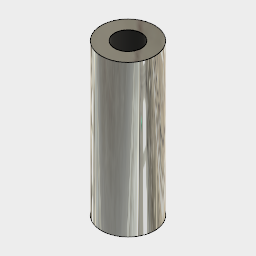
Print_Head_v5 (Autodesk Fusion 360 archive; units mm, degrees)
design "LM6LUU"
Autodesk Fusion 360 part; units mm, degrees
note: some values were not read from the file. Chosen so that the rebuilt part matches the saved one: which face or edge a step refers to. Set by a fixed rule: which sketch regions a step uses.
sketch "Sketch1" plane through (0, 0, 0) normal (0, 0, 1) x (1, 0, 0) in component "LM6LUU"
  circle A0 centre (0, 0) radius 6
  circle A1 centre (0, 0) radius 3
  dimension "d1" = 12
  dimension "d2" = 6
  measures "d1" diameter of A0
  measures "d2" diameter of A1
extrude "Extrude1" add sketch "Sketch1" along normal blind 34 makes body 1 in component "LM6LUU"
copy_body "CutPasteBodies1" bodies 1 removing the originals makes body 2 in component "LM6LUU"
component "LM6LUU" placed x (1, 0, 0) y (0, 1, 0) z (0, 0, 1) at (0, 0, 0)

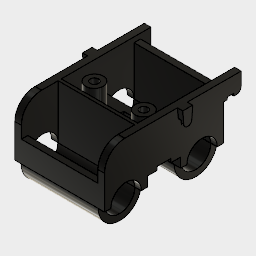
design "X Carriage"
Autodesk Fusion 360 part; units mm, degrees
sketch "Back" plane through (0, 0, 0) normal (0, 0, 1) x (1, 0, 0) in component "X Carriage"
  line L0 (17.75, 23.5) -> (-17.75, 23.5) construction
  line L1 (-17.75, 23.5) -> (-17.75, -23.5)
  line L2 (-17.75, -23.5) -> (17.75, -23.5)
  line L3 (17.75, -23.5) -> (17.75, 23.5)
  line L4 (0, 23.5) -> (0, -23.5) construction
  line L5 (-17.75, 23.5) -> (-17.75, 27.7)
  line L6 (-17.75, 27.7) -> (-15.1, 27.7)
  line L7 (17.75, 23.5) -> (17.75, 30.5)
  line L8 (17.75, 30.5) -> (15.1, 30.5)
  line L9 (15.1, 30.5) -> (15.1, 23.5)
  line L10 (-15.1, 27.7) -> (-15.1, 23.5)
  line L11 (-15.1, 23.5) -> (15.1, 23.5)
  line L12 (-15.1, 21) -> (15.1, 21)
  line L13 (15.1, 21) -> (15.1, -6.5)
  line L14 (15.1, -6.5) -> (-15.1, -6.5)
  line L15 (-15.1, -6.5) -> (-15.1, 21)
  line L16 (-15.1, -9) -> (15.1, -9)
  line L17 (15.1, -9) -> (15.1, -23.5)
  line L18 (-15.1, -9) -> (-15.1, -23.5)
  line L19 (15.1, -21) -> (-15.1, -21)
  line L20 (-9.75, 0) -> (9.75, 0) construction
  circle A0 centre (-9.75, 0) radius 1.6
  circle A1 centre (9.75, 0) radius 1.6
  circle A2 centre (-9.75, 0) radius 3.5
  circle A3 centre (9.75, 0) radius 3.5
  line L21 (15.1, -7.75) -> (-15.1, -7.75)
  line L22 (-15.1, -7.75) -> (-15.1, -6.5)
  line L23 (15.1, -7.75) -> (15.1, -6.5)
  line L24 (17.75, 9.2) -> (19.75, 9.2)
  line L25 (19.75, 9.2) -> (19.75, 5.3)
  line L26 (19.75, 5.3) -> (17.75, 5.3)
  line L27 (-17.75, 9.2) -> (-19.75, 9.2)
  line L28 (-19.75, 9.2) -> (-19.75, 5.3)
  line L29 (-19.75, 5.3) -> (-17.75, 5.3)
  line L30 (-4.5, -2.7) -> (4.5, -2.7)
  line L31 (4.5, -2.7) -> (4.5, 6.3)
  line L32 (4.5, 6.3) -> (-4.5, 6.3)
  line L33 (-4.5, 6.3) -> (-4.5, -2.7)
  line L34 (-3, -2.7) -> (-3, 3.3)
  line L35 (-3, 3.3) -> (3, 3.3)
  line L36 (3, 3.3) -> (3, -2.7)
  circle A4 centre (9.75, 0) radius 2.7
  circle A5 centre (-9.75, 0) radius 2.7
  line L37 (-15.1, 21) -> (-15.1, 23.5)
  line L38 (15.1, 21) -> (15.1, 23.5)
  line L39 (-15.1, 9) -> (15.1, 9)
  point P0 (0, 21)
  point P1 (0, -2.7)
  point P2 (0, 3.3)
  dimension "d1" = 35.5
  dimension "d2" = 47
  dimension "d3" = 4.2
  dimension "d5" = 7
  dimension "d7" = 30.2
  dimension "d8" = 27.5
  dimension "d9" = 2.5
  dimension "d10" = 2.5
  dimension "d11" = 2.5
  dimension "d12" = 19.5
  dimension "d13" = 3.2
  dimension "d14" = 3.2
  dimension "d15" = 7
  dimension "d16" = 7
  dimension "d17" = 21
  dimension "d18" = 1.25
  dimension "d20" = 3.9
  dimension "d21" = 2
  dimension "d22" = 28.8
  dimension "d23" = 9
  dimension "d24" = 9
  dimension "d25" = 6
  dimension "d26" = 6
  dimension "d27" = 5.4
  dimension "d28" = 5.4
  dimension "d37" = 12
  measures "d1" distance of L0.start L0.end
  measures "d2" distance of L0.start L2.end
  measures "d3" distance of L0.end L5.end
  measures "d5" distance of L0.start L7.end
  measures "d7" distance of L12.start L12.end
  measures "d8" distance of L12.start L14.end
  measures "d9" distance of L11 L12
  measures "d10" distance of L14 L16
  measures "d11" distance of L2 L19
  measures "d12" distance of L20.start L20.end
  measures "d13" diameter of A0
  measures "d14" diameter of A1
  measures "d15" diameter of A2
  measures "d16" diameter of A3
  measures "d17" distance of L12 L20
  measures "d18" distance of L16 L21
  measures "d20" distance of L24.end L25.end
  measures "d21" distance of L24.start L24.end
  measures "d22" distance of L2.end L26
  measures "d23" distance of L30.start L32.end
  measures "d24" distance of L30.start L30.end
  measures "d25" distance of L34.end L35.end
  measures "d26" distance of L34.start L34.end
  measures "d27" diameter of A4
  measures "d28" diameter of A5
  measures "d37" distance of L12 L39
extrude "Extrude1" add sketch "Back" along normal blind 21.25 contours L1 L2 L3 L5 L6 L7 L8 L9 L10 L13 L15 L16 L17 L18 L21 L22 L23 L37 L38 makes body 1 in component "X Carriage"
extrude "Extrude2" add sketch "Back" along normal blind 19.25 contours L11 L12 L37 L38 | L14 L21 L22 L23 | A2 | A3 | A4 | A5 bodies 1 makes body 2 at (13.2326, -0.3485, 12.8333) makes body 3 at (-6.2674, -0.3485, 12.8333) in component "X Carriage"
extrude "Extrude3" add sketch "Back" along normal blind 8.5 contours L2 L17 L18 L19 bodies 1 in component "X Carriage"
extrude "Extrude4" add sketch "Back" along normal blind 8.45 contours L13 L14 L15 L39 | L30 L34 L35 L36 bodies 1 2 3 in component "X Carriage"
sketch "Side" plane through (17.75, 0, 0) normal (1, 0, 0) x (0, 1, 0) in component "X Carriage"
  line L0 (-23.5, 0) -> (30.5, 0) construction
  line L1 (30.5, 21.25) -> (-23.5, 21.25) construction
  line L2 (-23.5, 21.25) -> (-23.5, 0) construction
  circle A0 centre (15, 0) radius 6
  circle A1 centre (-15, 0) radius 6
  circle A2 centre (-15, 0) radius 8.5
  circle A3 centre (15, 0) radius 8.5
  line L3 (23.5, 0) -> (23.5, 19.25) construction
  line L4 (9, 8.45) -> (-6.5, 8.45) construction
  line L5 (9, 0) -> (9, 8.45) construction
  line L6 (-9, 0) -> (-9, 21.25) construction
  line L7 (-6.5, 8.45) -> (-6.5, 19.25) construction
  line L8 (-6.5, 0) -> (-6.5, 3.8)
  line L9 (6.5, 0) -> (6.5, 3.8)
  line L10 (-6.5, 3.8) -> (6.5, 3.8)
  line L11 (-6.5, 0) -> (6.5, 0)
  line L12 (-2.7, 3.8) -> (-2.7, 5.25)
  line L13 (-2.7, 5.25) -> (2.7, 5.25)
  line L14 (2.7, 5.25) -> (2.7, 3.8)
  line L15 (0, 5.25) -> (0, 3.8) construction
  line L16 (-23.5, 0) -> (23.5, 0)
  line L17 (30.5, 21.25) -> (30.5, 16.1)
  line L18 (28.5, 14.1) -> (23.5, 14.1) construction
  line L19 (25, 15.1) -> (27.5, 15.1)
  line L20 (23.5, 14.1) -> (25, 14.1)
  line L21 (25, 14.1) -> (25, 15.1)
  line L22 (27.5, 15.1) -> (27.5, 14.1)
  line L23 (30.5, 14.1) -> (27.5, 14.1) construction
  arc A4 (28.5, 14.1) -> (30.5, 16.1) centre (28.5, 16.1) ccw
  line L24 (30.5, 16.1) -> (30.5, 0)
  line L25 (30.5, 0) -> (23.5, 0)
  line L26 (23.5, 0) -> (23.5, 14.1)
  line L27 (28.5, 14.1) -> (27.5, 14.1)
  line L28 (30.5, 0) -> (30.5, 21.25)
  dimension "d38" = 12
  dimension "d39" = 12
  dimension "d40" = 17
  dimension "d41" = 17
  dimension "d42" = 30
  dimension "d43" = 3.8
  dimension "d44" = 3.8
  dimension "d45" = 1.45
  dimension "d46" = 13
  dimension "d47" = 5.4
  dimension "d48" = 7.15
  dimension "d49" = 2.5
  dimension "d50" = 1.5
  dimension "d51" = 1
  dimension "d52" = 7
  dimension "d53" = 2
  measures "d38" diameter of A0
  measures "d39" diameter of A1
  measures "d40" diameter of A2
  measures "d41" diameter of A3
  measures "d42" distance of A0.centre A1.centre
  measures "d43" distance of L8.start L8.end
  measures "d44" distance of L9.start L9.end
  measures "d45" distance of L12.start L12.end
  measures "d46" distance of L8.end L9.end
  measures "d47" distance of L12.end L13.end
  measures "d48" distance of L1.start L23.start
  measures "d49" distance of L19.start L19.end
  measures "d50" distance of L18.end L20.end
  measures "d51" distance of L19.start L20.end
  measures "d52" distance of L3.end L1.start
  measures "d53" radius of A4
extrude "Extrude5" cut sketch "Side" against normal blind 35.5 contours A0 L16 | A0 L16 | L8 L9 L10 L11 L16 | A1 L16 | A1 L16 bodies 1 in component "X Carriage"
extrude "Extrude6" add sketch "Side" along normal blind -33 and the other way blind 2.5 contours A0 A3 L16 | A1 A2 L16 picked at (22.635, -0.4223) picked at (-7.3873, -0.7204) bodies 1 in component "X Carriage"
extrude "Extrude7" cut sketch "Side" against normal blind 2.65 contours L19 L20 L21 L22 A4 L24 L25 L26 L27 L28 bodies 1 in component "X Carriage"
fillet "Fillet1" radius 2 1 edges at (-16.425, 27.7, 0) on bodies 1 in component "X Carriage"
fillet "Fillet2" radius 8 3 edges at (16.425, -23.5, 21.25) (-16.425, -23.5, 21.25) (16.425, -23.5, 21.25) on bodies 1 in component "X Carriage"
extrude "Extrude8" cut sketch "Side" against normal blind 14 contours L10 L12 L13 L14 bodies 1 in component "X Carriage"
extrude "Extrude9" cut sketch "Side" along normal blind 14 from surface at -35.5 contours L10 L12 L13 L14 bodies 1 in component "X Carriage"
extrude "Extrude10" cut sketch "Back" along normal blind 3 from surface at 5.25 contours A4 | A5 bodies 1 in component "X Carriage"
sketch "Belt Catch" plane through (0, 3.3, 0) normal (0, 1, 0) x (-1, 0, 0) in component "X Carriage"
  line L0 (-3, 3.8) -> (3, 3.8)
  line L1 (3, 3.8) -> (3, 8.45)
  line L2 (3, 8.45) -> (-3, 8.45)
  line L3 (-3, 8.45) -> (-3, 3.8)
  line L4 (-3, 8.45) -> (3, 8.45)
  line L5 (-3, 3.8) -> (-3, 8.45)
  line L6 (3, 3.8) -> (3, 8.45)
  line L7 (-3, 3.8) -> (3, 3.8)
  line L8 (-3, 6.45) -> (3, 6.45)
  line L9 (0, 6.45) -> (0, 8.45) construction
  line L10 (-0.375, 6.45) -> (-0.375, 7.075)
  line L11 (-0.375, 7.075) -> (0.375, 7.075) construction
  line L12 (0.375, 7.075) -> (0.375, 6.45)
  arc A0 (0.375, 7.075) -> (-0.375, 7.075) centre (0, 7.075) ccw
  line L13 (-1.625, 7.075) -> (-1.625, 6.45)
  arc A1 (-1.625, 7.075) -> (-2.375, 7.075) centre (-2, 7.075) ccw
  line L14 (-2.375, 6.45) -> (-2.375, 7.075)
  line L15 (2.375, 7.075) -> (2.375, 6.45)
  arc A2 (2.375, 7.075) -> (1.625, 7.075) centre (2, 7.075) ccw
  line L16 (1.625, 6.45) -> (1.625, 7.075)
  point P0 (0, 7.075)
  dimension "d72" = 2
  dimension "d73" = 0.625
  dimension "d74" = 0.75
  dimension "d77" = 2
  dimension "d78" = 0
  measures "d72" distance of L2 L8
  measures "d73" distance of L10.start L10.end
  measures "d74" distance of L10.end L11.end
extrude "Extrude11" cut sketch "Belt Catch" against normal blind 6 contours L1 L2 L3 L4 L5 L6 L8 L10 L12 A0 L13 A1 L14 L15 A2 L16 bodies 1 in component "X Carriage"
sketch "Sping Catch" plane through (-17.75, 0, 0) normal (-1, 0, 0) x (0, -1, 0) in component "X Carriage"
  line L0 (-2.7, 3.8) -> (-2.7, 5.25)
  line L1 (-2.7, 5.25) -> (2.7, 5.25)
  line L2 (2.7, 5.25) -> (2.7, 3.8)
  line L3 (2.7, 3.8) -> (6.5, 3.8)
  line L4 (6.5, 3.8) -> (6.5, 0)
  line L5 (6.5, 0) -> (9, 0)
  arc A0 (21, 0) -> (9, 0) centre (15, 0) ccw
  line L6 (21, 0) -> (23.5, 0)
  line L7 (23.5, 0) -> (23.5, 13.25)
  arc A1 (23.5, 13.25) -> (15.5, 21.25) centre (15.5, 13.25) ccw
  line L8 (15.5, 21.25) -> (-27.7, 21.25)
  line L9 (-27.7, 21.25) -> (-27.7, 2)
  arc A2 (-27.7, 2) -> (-25.7, 0) centre (-25.7, 2) ccw
  line L10 (-25.7, 0) -> (-21, 0)
  arc A3 (-9, 0) -> (-21, 0) centre (-15, 0) ccw
  line L11 (-9, 0) -> (-6.5, 0)
  line L12 (-6.5, 0) -> (-6.5, 3.8)
  line L13 (-6.5, 3.8) -> (-2.7, 3.8)
  line L14 (-27.7, 2) -> (-27.7, 21.25)
  line L15 (-27.7, 21.25) -> (15.5, 21.25)
  line L16 (-9.2, 21.25) -> (-8.85, 16.45)
  line L17 (-8.85, 16.45) -> (-5.65, 16.45)
  line L18 (-5.65, 16.45) -> (-5.3, 21.25)
  line L19 (-9.2, 21.25) -> (-5.3, 21.25)
  line L20 (-7.25, 21.25) -> (-7.25, 16.45) construction
  arc A4 (-8.85, 16.45) -> (-5.65, 16.45) centre (-7.25, 16.5667) ccw
  line L21 (-5.3, 0) -> (-5.3, 21.25) construction
  line L22 (-9.2, 0) -> (-9.2, 21.25) construction
  arc A5 (-8.9229, 17.45) -> (-5.5771, 17.45) centre (-7.25, 18.3493) ccw
  point P0 (-9.2, 0)
  point P1 (-5.3, 0)
  dimension "d82" = 3.2
  dimension "d83" = 4.8
  dimension "d84" = 1.6026
  dimension "d91" = 3.9
  dimension "d92" = 1
  measures "d82" distance of L16.end L17.end
  measures "d83" distance of L20.start L20.end
  measures "d91" distance of L16.start L18.end
  measures "d92" distance of L17.end A5.end
extrude "Extrude12" add sketch "Sping Catch" along normal blind 2.1 contours L8 L15 L16 L18 L19 A5 | L16 L17 A5 | L17 L18 A5 | L17 A4 bodies 1 in component "X Carriage"
extrude "Extrude13" cut sketch "Sping Catch" along normal blind 1.1 contours L16 L17 A5 | L17 L18 A5 | L17 A4 bodies 1 in component "X Carriage"
mirror "Mirror1" about plane through (0, 0, 0) normal (1, 0, 0) of "Extrude12", "Extrude13" in component "X Carriage"
component "X Carriage" placed x (1, 0, 0) y (0, 1, 0) z (0, 0, 1) at (0, 0, 0)
equation "d31 = 21.25 mm - 2 mm"
equation "d35 = 21.25 mm - 12.8 mm"
equation "d56 = -35.50 mm + 2.5 mm"
equation "d73 = 1 mm - ( 0.75 / 2 ) * 1 mm"
